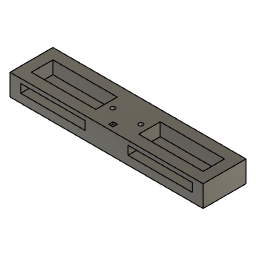
AttacheUp v3 (Autodesk Fusion 360 design; units mm, degrees)
Autodesk Fusion 360 part; units mm, degrees
sketch "Esquisse1" plane through (0, 0, 0) normal (0, 0, 1) x (1, 0, 0)
  line L0 (0, 0) -> (90, 0)
  line L1 (90, 0) -> (90, 20)
  line L2 (90, 20) -> (0, 20)
  line L3 (0, 20) -> (0, 0)
  circle A0 centre (38.5, 9.5) radius 1
  circle A1 centre (51.5, 9.5) radius 1
  dimension "d1" = 90
  dimension "d2" = 20
  dimension "d3" = 2
  dimension "d4" = 2
  dimension "d5" = 13
  dimension "d6" = 9.5
  dimension "d7" = 38.5
  dimension "d8" = 9.5
  constraint horizontal L0
  constraint vertical L1
  constraint horizontal L2
  constraint vertical L3
  constraint coincident L0.start L3.end
  measures "d1" distance of L1.end L2.end
  measures "d2" distance of L0.end L1.end
  measures "d3" diameter of A0
  measures "d4" diameter of A1
  measures "d5" distance of A0.centre A1.centre
  measures "d6" distance of L0 A1.centre
  measures "d7" distance of L1 A1.centre
  measures "d8" distance of L0 A0.centre
extrude "Extrusion1" add sketch "Esquisse1" along normal blind 10
sketch "Esquisse2" plane through (0, 0, 0) normal (0, -1, 0) x (1, 0, 0)
  line L0 (0, 0) -> (90, 0)
  line L1 (90, 0) -> (90, 10)
  line L2 (90, 10) -> (0, 10)
  line L3 (0, 10) -> (0, 0)
  line L4 (5, 8) -> (35, 8)
  line L5 (35, 8) -> (35, 4)
  line L6 (35, 4) -> (5, 4)
  line L7 (5, 4) -> (5, 8)
  line L8 (55, 8) -> (85, 8)
  line L9 (85, 8) -> (85, 4)
  line L10 (85, 4) -> (55, 4)
  line L11 (55, 4) -> (55, 8)
  dimension "d11" = 4
  dimension "d12" = 4
  dimension "d13" = 2
  dimension "d14" = 2
  dimension "d15" = 30
  dimension "d16" = 30
  dimension "d18" = 5
  dimension "d19" = 5
  constraint horizontal L4
  constraint vertical L5
  constraint horizontal L6
  constraint vertical L7
  constraint horizontal L8
  constraint vertical L9
  constraint horizontal L10
  constraint vertical L11
  measures "d11" distance of L4.end L5.end
  measures "d12" distance of L8.end L9.end
  measures "d13" distance of L2 L8
  measures "d14" distance of L2 L4
  measures "d15" distance of L8.start L8.end
  measures "d16" distance of L4.start L4.end
  measures "d18" distance of L1 L9
  measures "d19" distance of L3 L7
extrude "Extrusion2" cut sketch "Esquisse2" against normal blind 15 contours L4 L5 L6 L7 | L8 L9 L10 L11
sketch "Esquisse3" plane through (0, 0, 10) normal (0, 0, 1) x (-1, 0, 0)
  circle A0 centre (-38.5, -9.5) radius 1
  circle A1 centre (-51.5, -9.5) radius 1
  line L0 (0, -20) -> (0, 0)
  line L1 (0, 0) -> (-90, 0)
  line L2 (-90, 0) -> (-90, -20)
  line L3 (-90, -20) -> (0, -20)
  line L4 (-44, -4) -> (-46, -4)
  line L5 (-46, -4) -> (-46, -2)
  line L6 (-46, -2) -> (-44, -2)
  line L7 (-44, -2) -> (-44, -4)
  dimension "d22" = 2
  dimension "d23" = 2
  dimension "d24" = 2
  dimension "d25" = 44
  constraint horizontal L4
  constraint vertical L5
  constraint horizontal L6
  constraint vertical L7
  measures "d22" distance of L4.start L4.end
  measures "d23" distance of L4.end L5.end
  measures "d24" distance of L1 L6
  measures "d25" distance of L0 L7
extrude "Extrusion3" cut sketch "Esquisse3" against normal blind 1 contours L4 L5 L6 L7
sketch "Esquisse4" plane through (0, 0, 10) normal (0, 0, 1) x (-1, 0, 0)
  line L0 (-46, -4) -> (-46, -2)
  line L1 (-46, -2) -> (-44, -2)
  line L2 (-44, -2) -> (-44, -4)
  line L3 (-44, -4) -> (-46, -4)
  circle A0 centre (-38.5, -9.5) radius 1
  circle A1 centre (-51.5, -9.5) radius 1
  line L4 (0, -20) -> (0, 0)
  line L5 (0, 0) -> (-90, 0)
  line L6 (-90, 0) -> (-90, -20)
  line L7 (-90, -20) -> (0, -20)
  line L8 (-5, -15) -> (-35, -15)
  line L9 (-35, -15) -> (-35, -5)
  line L10 (-35, -5) -> (-5, -5)
  line L11 (-5, -5) -> (-5, -15)
  line L12 (-55, -15) -> (-85, -15)
  line L13 (-85, -15) -> (-85, -5)
  line L14 (-85, -5) -> (-55, -5)
  line L15 (-55, -5) -> (-55, -15)
  dimension "d28" = 10
  dimension "d29" = 10
  dimension "d30" = 5
  dimension "d31" = 5
  dimension "d32" = 30
  dimension "d33" = 5
  dimension "d34" = 5
  dimension "d35" = 30
  constraint horizontal L8
  constraint vertical L9
  constraint horizontal L10
  constraint vertical L11
  constraint horizontal L12
  constraint vertical L13
  constraint horizontal L14
  constraint vertical L15
  measures "d28" distance of L8.start L10.end
  measures "d29" distance of L12.end L13.end
  measures "d30" distance of L5 L10
  measures "d31" distance of L5 L14
  measures "d32" distance of L9.end L10.end
  measures "d33" distance of L4 L11
  measures "d34" distance of L6 L13
  measures "d35" distance of L13.end L14.end
extrude "Extrusion4" cut sketch "Esquisse4" against normal blind 5 contours L8 L9 L10 L11 | L12 L13 L14 L15
